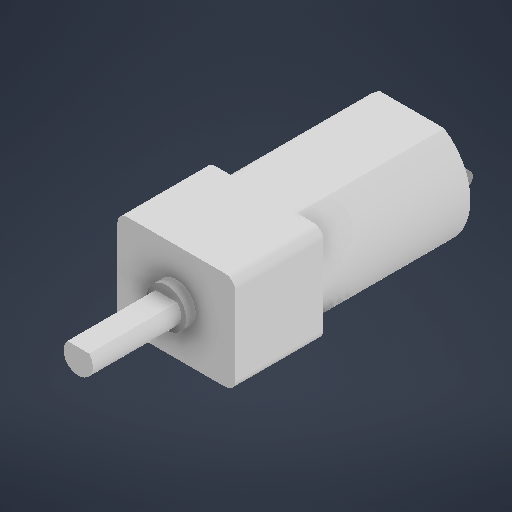
# Autodesk Inventor part: Мотор 15x12x10 с редуктоом
Saved by Autodesk Inventor 2026.2 (Build 302298000, 298)
## iProperties
Created: 2026-03-05
Part Number: Мотор 15x12x10 с редуктоом
Material: Типовые
Document SubType Name: Modeling
Designer: Leonid
Density: 1 g/cm^3
Appearance: По умолчанию
Author: Leonid
Autodesk Inventor part; units mm, degrees
ref_plane "YZ Plane" through (0, 0, 0) normal (1, 0, 0) x (0, 1, 0)
ref_plane "XZ Plane" through (0, 0, 0) normal (0, 1, 0) x (-1, 0, 0)
ref_plane "XY Plane" through (0, 0, 0) normal (0, 0, 1) x (1, 0, 0)
sketch "Эскиз2" plane through (0, 0, 0) normal (0, 0, 1) x (1, 0, 0)
  line L0 (-5, -5) -> (5, -5)
  line L1 (6, -4) -> (6, 4)
  line L2 (5, 5) -> (-5, 5)
  line L3 (-6, 4) -> (-6, -4)
  line L4 (-6, -5) -> (6, 5) construction
  line L5 (6, -5) -> (-6, 5) construction
  arc A0 (-5, 5) -> (-6, 4) centre (-5, 4) ccw
  arc A1 (6, 4) -> (5, 5) centre (5, 4) ccw
  arc A2 (5, -5) -> (6, -4) centre (5, -4) ccw
  arc A3 (-6, -4) -> (-5, -5) centre (-5, -4) ccw
  arc A4 (-3.3166, 5) -> (-3.3166, -5) centre (0, 0) ccw
  arc A5 (3.3166, -5) -> (3.3166, 5) centre (0, 0) ccw
  dimension "d0" = 12
  dimension "d1" = 10
  dimension "d2" = 1
  constraints: 12 end point, 12 point on circle, 12 point on line, 10 tangent, 6 centre point, 3 equal radius, 2 midpoint, 2 parallel, 1 coincident, 1 horizontal, 1 perpendicular
  measures "d0" distance of L5.end L4.end
  measures "d1" distance of L4.end L5.start
  measures "d2" radius of A0
extrude "Выдавливание1" add sketch "Эскиз2" against normal blind 15 contours A4 L2 A5 L0
extrude "Выдавливание2" add sketch "Эскиз2" along normal blind 9
sketch "Эскиз3" plane through (0, 0, 9) normal (0, 0, 1) x (1, 0, 0)
  arc A0 (-1.118, 1) -> (1.118, 1) centre (0, 0) ccw
  circle A1 centre (0, 0) radius 2
  line L0 (-1.118, 1) -> (1.118, 1)
  arc A2 (1.118, 1) -> (-1.118, 1) centre (0, 0) ccw construction
  dimension "d8" = 3
  dimension "d9" = 4
  dimension "d10" = 2.5
  constraints: 4 point on circle, 3 centre point, 2 coincident, 2 end point, 1 horizontal
  measures "d8" diameter of A0
  measures "d9" diameter of A1
extrude "Выдавливание3" add sketch "Эскиз3" along normal blind 1 contours L0 A0 | A1
extrude "Выдавливание4" add sketch "Эскиз3" along normal blind 10 contours L0 A0
sketch "Эскиз4" plane through (0, 0, -15) normal (0, 0, -1) x (-1, 0, 0)
  circle A0 centre (0, 0) radius 2.5
  line L0 (-4, 0.75) -> (-3.5, 0.75)
  line L1 (-3.5, 0.75) -> (-3.5, -0.75)
  line L2 (-3.5, -0.75) -> (-4, -0.75)
  line L3 (-4, -0.75) -> (-4, 0.75)
  line L4 (3.5, 0.75) -> (4, 0.75)
  line L5 (4, 0.75) -> (4, -0.75)
  line L6 (4, -0.75) -> (3.5, -0.75)
  line L7 (3.5, -0.75) -> (3.5, 0.75)
  line L8 (-3.5, 0) -> (3.5, 0) construction
  dimension "d15" = 5
  dimension "d18" = 8
  dimension "d19" = 7
  dimension "d20" = 1.5
  constraints: 18 end point, 4 parallel, 3 horizontal, 3 midpoint, 2 coincident, 2 equal length, 2 perpendicular, 1 centre point
  measures "d15" diameter of A0
  measures "d18" distance between parallel lines of L5 L3
  measures "d19" distance between parallel lines of L7 L1
  measures "d20" distance of L4.end L5.end
extrude "Выдавливание5" add sketch "Эскиз4" along normal blind 1.75 contours A0
extrude "Выдавливание6" add sketch "Эскиз4" along normal blind 2.25 contours L0 L1 L2 L3 | L4 L5 L6 L7
fillet "Сопряжение1" radius 0.75 4 edges at (3.75, 0.75, -17.25) (3.75, -0.75, -17.25) (-3.75, 0.75, -17.25) (-3.75, -0.75, -17.25)
